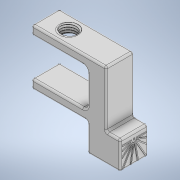
# Autodesk Inventor part: clamp-02
Saved by Autodesk Inventor 2020 (Build 240168000, 168)
## iProperties
Created: 2020-05-22
Part Number: clamp-02
Material: Generic
Document SubType Name: Modeling
Designer: alejandrosalazar
Density: 1 g/cm^3
Appearance: Default
Author: alejandrosalazar
Autodesk Inventor part; units mm, degrees
ref_plane "YZ Plane" through (0, 0, 0) normal (1, 0, 0) x (0, 1, 0)
ref_plane "XZ Plane" through (0, 0, 0) normal (0, 1, 0) x (-1, 0, 0)
ref_plane "XY Plane" through (0, 0, 0) normal (0, 0, 1) x (1, 0, 0)
sketch "Sketch2" plane through (0, 0, 0) normal (1, 0, 0) x (0, 1, 0)
  line L0 (0, 0) -> (60, 0)
  line L1 (60, 0) -> (60, -30)
  line L2 (60, -30) -> (0, -30)
  line L3 (0, -30) -> (0, 0)
  dimension "d0" = 60
  dimension "d1" = 30
  constraints: 8 end point, 2 parallel, 1 horizontal, 1 perpendicular
  measures "d0" distance of L1.end L2.end
  measures "d1" distance of L0.end L1.end
extrude "Extrusion1" add sketch "Sketch2" along normal blind 80
sketch "Sketch3" plane through (0, 0, 0) normal (0, 0, 1) x (1, 0, 0)
  line L0 (0, 60) -> (0, 0) projected
  line L1 (0, 10) -> (60, 10)
  line L2 (60, 10) -> (60, 50)
  line L3 (60, 50) -> (0, 50)
  line L4 (0, 50) -> (0, 10)
  dimension "d4" = 60
  dimension "d5" = 40
  constraints: 8 end point, 2 parallel, 1 horizontal, 1 perpendicular, 1 point on line
  measures "d4" distance of L3.end L2.end
  measures "d5" distance of L2.end L1.end
extrude "Extrusion2" cut sketch "Sketch3" against normal blind 80
sketch "Sketch4" plane through (80, 0, 0) normal (1, 0, 0) x (0, 0, -1)
  line L0 (0, 0) -> (30, 0) projected
  line L1 (5, 0) -> (25, 0)
  line L2 (25, 0) -> (25, -30)
  line L3 (25, -30) -> (5, -30)
  line L4 (5, -30) -> (5, 0)
  dimension "d8" = 20
  dimension "d9" = 30
  constraints: 8 end point, 2 parallel, 1 horizontal, 1 perpendicular, 1 point on line
  measures "d8" distance of L2.end L3.end
  measures "d9" distance of L1.end L2.end
extrude "Extrusion3" add sketch "Sketch4" against normal blind 20
sketch "Sketch5" plane through (0, 60, 0) normal (0, 1, 0) x (1, 0, 0)
  circle A0 centre (25, 15) radius 10
  point P0 (0, 0)
  dimension "d12" = 20
  constraints: 1 centre point
  measures "d12" diameter of A0
extrude "Extrusion4" cut sketch "Sketch5" against normal blind 10
fillet "Fillet1" radius 5 2 edges at (60, 50, -15) (60, 10, -15)
sketch "Sketch23" plane through (80, 0, 0) normal (1, 0, 0) x (0, 0, -1)
  line L0 (25, 0) -> (25, -30) projected
  line L1 (0, 0) -> (5, 0) projected
  line L2 (25, -30) -> (5, -30)
  line L3 (5, -30) -> (5, 0)
  line L4 (5, 0) -> (25, 0)
  line L5 (25, 0) -> (25, -30)
  constraints: 8 end point, 2 parallel, 1 horizontal, 1 perpendicular
extrude "Extrusion12" add sketch "Sketch23" along normal blind 15
sketch "Sketch24" plane through (60, -30, -5) normal (0, 0, 1) x (1, 0, 0)
  line L0 (35, 30) -> (35, 0) projected
  line L1 (0, 30) -> (0, 0) projected
  line L2 (35, 30) -> (0, 30)
  line L3 (0, 30) -> (0, 0)
  line L4 (0, 0) -> (35, 0)
  line L5 (35, 0) -> (35, 30)
  point P0 (-60, 30)
  constraints: 8 end point, 2 parallel, 1 horizontal, 1 perpendicular
extrude "Extrusion13" add sketch "Sketch24" along normal blind 5
sketch "Sketch25" plane through (60, -30, -25) normal (0, 0, -1) x (-1, 0, 0)
  line L0 (-20, 30) -> (-35, 30) projected
  line L1 (-35, 30) -> (0, 30)
  line L2 (0, 30) -> (0, 0)
  line L3 (0, 0) -> (-35, 0)
  line L4 (-35, 0) -> (-35, 30)
  point P0 (60, 30)
  constraints: 8 end point, 2 parallel, 1 horizontal, 1 perpendicular
extrude "Extrusion14" add sketch "Sketch25" along normal blind 5
thread "Thread8" size "M20x2.5" class "6H" standard "ANSI Metric M Profile" length 10
sketch "Sketch30" plane through (25, 50, -15) normal (-1, 0, 0) x (0, 0, 1)
  line L0 (10, 0) -> (10, 10)
  line L1 (10, 10) -> (8.1463, 10)
  line L2 (8.1463, 10) -> (8.1463, 0)
  line L3 (8.1463, 0) -> (10, 0)
  line L4 (0, -105.71) -> (0, 29.285) projected
  constraints: 8 end point
revolve "Revolution4" add sketch "Sketch30" angle 360 about axis through (25, 50, -15) along (0, 1, 0) separate body
sketch "Sketch29" plane through (25, 50, -5) normal (1, 0, 0) x (0, 1, 0)
  line L0 (-1.4584, -0.1266) -> (-1.2501, -0.1266) construction
  line L1 (0.2082, -1.7274) -> (-0.0001, -2.1276) construction
  line L2 (-2.5001, -2.1276) -> (-2.7084, -1.7274) construction
  line L3 (-1.0418, -0.1266) -> (-1.2501, 0.2736) construction
  line L4 (-1.2501, 0.2736) -> (-1.4584, -0.1266) construction
  line L5 (-2.5001, -2.1276) -> (-2.2918, -1.7274) construction
  line L6 (-1.0418, -0.1266) -> (-0.2084, -1.7274)
  line L7 (-2.7084, -1.7274) -> (-2.2918, -1.7274) construction
  arc A0 (-2.7084, -1.7274) -> (-2.5001, -1.8538) centre (-2.5001, -1.6189) ccw construction
  line L8 (0.2082, -1.7274) -> (-0.2084, -1.7274) construction
  line L9 (-2.5001, -2.1276) -> (-2.5001, -1.7274) construction
  line L10 (-0.0001, -2.1276) -> (-0.0001, -1.7274) construction
  line L11 (-1.2501, 0.2736) -> (-1.2501, -0.0002) construction
  line L12 (-2.5001, -1.8538) -> (-0.0001, -1.8538)
  arc A1 (-2.5001, -1.8538) -> (-2.2918, -1.7274) centre (-2.5001, -1.6189) ccw
  line L13 (-0.2084, -1.7274) -> (-0.0001, -2.1276) construction
  line L14 (-2.2918, -1.7274) -> (-1.4584, -0.1266)
  line L15 (-0.0001, -0.0002) -> (-0.0001, 0.0177)
  line L16 (-0.0001, 0.0177) -> (-0.0001, -0.0002)
  line L17 (-0.0001, -0.0002) -> (0.0334, -0.0002)
  arc A2 (-0.2084, -1.7274) -> (-0.0001, -1.8538) centre (-0.0001, -1.6189) ccw
  arc A3 (-0.0001, -1.8538) -> (0.2082, -1.7274) centre (-0.0001, -1.6189) ccw construction
  arc A4 (-1.2501, -0.0002) -> (-1.4584, -0.1266) centre (-1.2501, -0.235) ccw
  arc A5 (-1.0418, -0.1266) -> (-1.2501, -0.0002) centre (-1.2501, -0.235) ccw
  line L18 (-1.2501, -0.0002) -> (-1.2501, -0.1266) construction
  line L19 (-1.2501, -0.1266) -> (-1.0418, -0.1266) construction
  dimension "d105" = 55
  dimension "d106" = 0.4002
  dimension "d107" = 0.4002
  dimension "Sketch29_ThreadOffset" = 0
  dimension "Sketch29_MajorRadius" = 1.8537
  dimension "d110" = 2.5
  dimension "Sketch29_MinorRadius" = 0
  constraints: 40 end point, 12 point on circle, 10 parallel, 8 tangent, 6 centre point, 6 collinear, 2 midpoint, 2 point on line, 1 horizontal, 1 perpendicular, 3 other
  measures "d105" angle of L6 L14
  measures "d106" distance of L3.end L0.end
  measures "d107" distance of L1.end L10.end
  measures "Sketch29_ThreadOffset" distance between parallel lines of L15 L10
  measures "Sketch29_MajorRadius" distance from line of L12 L15.start
  measures "d110" distance from line of L1.end L9
  measures "Sketch29_MinorRadius" distance edge to line of A5 L17
coil "Coil3" sketch "Sketch29" operation cut axis through (25, 50, -15) along (0, 1, 0) pitch 2.5025 turns 5.994006 hand right bodies 2
fillet "Fillet2" radius 2 38 edges at (80, 30, 0) (80, 60, -15) (40, 60, 0) (40, 60, -30) (0, 60, -15) (60, -15, 0) (77.5, -30, 0) (95, -15, 0) (95, -30, -15) (87.5, 0, 0) (95, 0, -15) (80, 0, -15) (87.5, 0, -30) (80, 30, -30) (95, -15, -30) (77.5, -30, -30) (60, -15, -30) (30, 0, -30) (58.5355, 48.5355, -30) (60, 30, -30) (58.5355, 11.4645, -30) (27.5, 10, -30) (27.5, 50, -30) (60, 0, -15) (60, -30, -15) (30, 0, 0) (0, 0, -15) (0, 5, 0) (0, 5, -30) (0, 10, -15) (58.5355, 11.4645, 0) (60, 30, 0) (58.5355, 48.5355, 0) (27.5, 50, 0) (27.5, 10, 0) (0, 50, -15) (0, 55, -30) (0, 55, 0)
sketch "Sketch49" plane through (60, 0, 0) normal (-1, 0, 0) x (0, 0, 1)
  line L0 (-15, -25) -> (-16.05, -25)
  line L1 (-16.05, -25) -> (-16.05, -23.95)
  line L2 (-16.05, -23.95) -> (-15, -23.95)
  line L3 (-15, -23.95) -> (-15, -25)
  line L4 (-15, -25) -> (-13.95, -25)
  line L5 (-13.95, -25) -> (-13.95, -23.95)
  line L6 (-13.95, -23.95) -> (-15, -23.95)
  line L7 (-15, -23.95) -> (-15, -25)
  line L8 (-15, -25) -> (-16.05, -25)
  line L9 (-16.05, -25) -> (-16.05, -26.05)
  line L10 (-16.05, -26.05) -> (-15, -26.05)
  line L11 (-15, -26.05) -> (-15, -25)
  line L12 (-15, -25) -> (-13.95, -25)
  line L13 (-13.95, -25) -> (-13.95, -26.05)
  line L14 (-13.95, -26.05) -> (-15, -26.05)
  line L15 (-15, -26.05) -> (-15, -25)
  point P0 (0, 0)
  dimension "d279" = 1.05
  dimension "d280" = 1.05
  dimension "d281" = 1.05
  dimension "d282" = 1.05
  dimension "d283" = 1.05
  dimension "d284" = 1.05
  dimension "d285" = 1.05
  dimension "d286" = 1.05
  constraints: 32 end point, 8 parallel, 4 horizontal, 4 perpendicular
  measures "d279" distance of L1.end L2.end
  measures "d280" distance of L0.end L1.end
  measures "d281" distance of L6.end L5.end
  measures "d282" distance of L5.end L4.end
  measures "d283" distance of L10.end L9.end
  measures "d284" distance of L9.end L8.end
  measures "d285" distance of L13.end L14.end
  measures "d286" distance of L12.end L13.end
extrude "Extrusion23" cut sketch "Sketch49" against normal blind 6.9 bodies 1
sketch "Sketch67" plane through (95, 0, 0) normal (1, 0, 0) x (0, 0, -1)
  circle A0 centre (15, -6.425) radius 1
  point P0 (0, 0)
  dimension "d1059" = 2
  constraints: 1 centre point
  measures "d1059" diameter of A0
extrude "Extrusion35" cut sketch "Sketch67" against normal blind 9 bodies 1
sketch "Sketch68" plane through (95, 0, 0) normal (1, 0, 0) x (0, 0, -1)
  line L0 (14.5, -36.425) -> (15, -36.425)
  line L1 (18.7861, -7.271) -> (46.0264, -17.1856)
  line L2 (15.5, -36.425) -> (15, -36.425)
  line L3 (14.5, -36.425) -> (15, -36.425)
  line L4 (18.2685, -8.5149) -> (40.475, -27.1483)
  line L5 (15.5, -36.425) -> (15, -36.425)
  line L6 (14.5, -36.425) -> (15, -36.425)
  line L7 (15.5, -36.425) -> (15, -36.425)
  line L8 (14.5, -36.425) -> (15, -36.425)
  line L9 (15.5, -36.425) -> (15, -36.425)
  line L10 (11.2139, -7.271) -> (-13.3618, -16.2158)
  line L11 (14.5, -36.425) -> (15, -36.425)
  line L12 (15.5, -36.425) -> (15, -36.425)
  line L13 (11.7315, -8.5149) -> (-8.3027, -25.3256)
  line L14 (14.5, -36.425) -> (15, -36.425)
  line L15 (15.5, -36.425) -> (15, -36.425)
  line L16 (14.5, -36.425) -> (15, -36.425)
  line L17 (15.5, -36.425) -> (15, -36.425)
  line L18 (14.5, -36.425) -> (15, -36.425)
  line L19 (15.5, -36.425) -> (15, -36.425)
  circle A0 centre (15, -6.425) radius 2.8794
  line L20 (11.5559, -8.2106) -> (-13.0198, -17.1555)
  line L21 (12.6434, -9.5067) -> (-0.433, -32.1558)
  line L22 (12.3743, -9.2809) -> (-7.6599, -26.0917)
  line L23 (13.8395, -10.1269) -> (9.2982, -35.8824)
  line L24 (13.5094, -10.0067) -> (0.433, -32.6558)
  line L25 (15.1756, -10.3005) -> (19.717, -36.0561)
  line L26 (14.8244, -10.3005) -> (10.283, -36.0561)
  line L27 (16.1605, -10.1269) -> (20.7018, -35.8824)
  line L28 (16.4906, -10.0067) -> (29.567, -32.6558)
  line L29 (17.6257, -9.2809) -> (37.6599, -26.0917)
  line L30 (17.3566, -9.5067) -> (30.433, -32.1558)
  line L31 (17.4936, -7.8647) -> (43.0198, -17.1555)
  line L32 (17.8356, -6.925) -> (47.8356, -6.925)
  line L33 (14.5, -36.425) -> (15, -36.425)
  line L34 (17.8356, -5.925) -> (47.8356, -5.925)
  line L35 (15.5, -36.425) -> (15, -36.425)
  line L36 (12.1644, -5.925) -> (-15, -5.925)
  line L37 (14.5, -36.425) -> (15, -36.425)
  line L38 (11.1529, -6.925) -> (-15, -6.925)
  line L39 (15.5, -36.425) -> (15, -36.425)
  arc A1 (11.1529, -6.925) -> (11.2139, -7.271) centre (15, -6.425) ccw
  arc A2 (11.5559, -8.2106) -> (11.7315, -8.5149) centre (15, -6.425) ccw
  arc A3 (12.3743, -9.2809) -> (12.6434, -9.5067) centre (15, -6.425) ccw
  arc A4 (13.5094, -10.0067) -> (13.8395, -10.1269) centre (15, -6.425) ccw
  arc A5 (14.8244, -10.3005) -> (15.1756, -10.3005) centre (15, -6.425) ccw
  arc A6 (16.1605, -10.1269) -> (16.4906, -10.0067) centre (15, -6.425) ccw
  arc A7 (17.3566, -9.5067) -> (17.6257, -9.2809) centre (15, -6.425) ccw
  arc A8 (18.2685, -8.5149) -> (18.4441, -8.2106) centre (15, -6.425) ccw
  arc A9 (18.7861, -7.271) -> (11.1529, -5.925) centre (15, -6.425) ccw
  line L40 (2, -2) -> (2, -28) projected
  line L41 (2, -5.925) -> (2, -6.925)
  line L42 (2, -10.6245) -> (2, -11.6887)
  line L43 (2, -16.6806) -> (2, -17.986)
  line L44 (2, -28) -> (3.121, -28)
  line L45 (2, -28) -> (28, -28) projected
  line L46 (10.688, -28) -> (11.7035, -28)
  line L47 (18.2965, -28) -> (19.312, -28)
  line L48 (26.879, -28) -> (28.0337, -28)
  line L49 (28, -28) -> (28, -2) projected
  line L50 (28, -17.986) -> (28, -16.6806)
  line L51 (28, -11.6887) -> (28, -10.6245)
  line L52 (28, -6.925) -> (28, -5.925)
  point P0 (0, 0)
  point P1 (2, -27.9417)
  point P2 (28, -27.9417)
  point P3 (18.8471, -6.925)
  dimension "d1069" = 30
  dimension "d1074" = 30
  dimension "d1110" = 30
  dimension "d1113" = 30
  constraints: 100 end point, 40 point on line, 22 point on circle, 10 centre point, 1 coincident
  measures "d1069" distance of L32.start L1.end
  measures "d1074" distance of L31.start L4.end
  measures "d1110" distance of L32.end L32.start
  measures "d1113" distance of L34.start L34.end
extrude "Extrusion36" add sketch "Sketch68" along normal blind 0.7 contours L1 L49 L31 A0 L32 A9 | A9 L34 L49 L32 | L32 A0 L34 A9 | A8 L4 L49 L29 A7 L30 L45 L28 A6 L27 L25 A5 L26 L23 A4 L24 L44 L40 L21 A3 L22 L13 A2 L20 L10 A1 L38 L36 A0 L31 bodies 1
equation "\"d105\" = d112"
equation "\"d106\" = 0.160083 * Sketch29_Pitch"
equation "\"d107\" = 0.160083 * Sketch29_Pitch"
equation "\"d110\" = Sketch29_Pitch"
equation "\"d55\" = 55deg"
equation "\"Sketch15_Pitch\" = 0.5"
equation "\"d76\" = 55deg"
equation "\"Sketch18_Pitch\" = 2.5"
equation "\"d112\" = 55deg"
equation "\"Sketch29_Pitch\" = 2.5"
equation "\"d141\" = 55deg"
equation "\"Sketch33_Pitch\" = 0.7"
equation "\"d166\" = 55deg"
equation "\"Sketch36_Pitch\" = 0.5"
equation "\"d186\" = 55deg"
equation "\"Sketch38_Pitch\" = 0.8"
equation "\"d207\" = 55deg"
equation "\"Sketch40_Pitch\" = 0.5"
equation "\"d227\" = 55deg"
equation "\"Sketch42_Pitch\" = 0.5"
equation "\"d250\" = 55deg"
equation "\"Sketch45_Pitch\" = 0.5"
body "Solid1"
body "Solid4"
